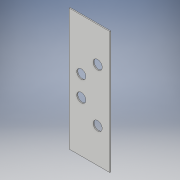
# Autodesk Inventor part: Holding Plate
Saved by Autodesk Inventor 2018 (Build 220112000, 112)
## iProperties
Created: 2019-01-15
Part Number: Holding Plate
Material: Generic
Document SubType Name: Modeling
Designer: Gabriel
Density: 1 g/cm^3
Appearance: Default
Author: Gabriel
Autodesk Inventor part; units mm, degrees
ref_plane "YZ Plane" through (0, 0, 0) normal (1, 0, 0) x (0, 1, 0)
ref_plane "XZ Plane" through (0, 0, 0) normal (0, 1, 0) x (-1, 0, 0)
ref_plane "XY Plane" through (0, 0, 0) normal (0, 0, 1) x (1, 0, 0)
sketch "Sketch1" plane through (0, 0, 0) normal (0, 0, 1) x (1, 0, 0)
  line L0 (-52.0393, 256.0699) -> (74.9607, 256.0699)
  line L1 (74.9607, 256.0699) -> (74.9607, -124.9301)
  line L2 (74.9607, -124.9301) -> (-52.0393, -124.9301)
  line L3 (-52.0393, -124.9301) -> (-52.0393, 256.0699)
  point P0 (0, 0)
  dimension "d0" = 127
  dimension "d1" = 381
  constraints: 8 end point, 2 parallel, 1 horizontal, 1 perpendicular
  measures "d0" distance of L1.end L2.end
  measures "d1" distance of L0.end L1.end
extrude "Extrusion1" add sketch "Sketch1" along normal blind 3.175
sketch "Sketch3" plane through (0, 0, 3.175) normal (0, 0, 1) x (1, 0, 0)
  line L0 (-52.0393, 256.0699) -> (-52.0393, -124.9301) projected
  line L1 (-52.0393, 65.5699) -> (-45.6893, 65.5699) construction
  line L2 (-45.6893, 65.5699) -> (-13.9457, 64.9297) construction
  line L3 (-13.9457, 64.9297) -> (-13.9457, 96.6797) construction
  line L4 (-13.9457, 64.9297) -> (17.8043, 64.9297) construction
  line L5 (-13.9457, 64.9297) -> (-13.9457, 33.1797) construction
  line L6 (-13.9457, 64.9297) -> (17.8043, 64.9297) construction
  line L7 (-13.9457, 96.6797) -> (36.8543, 96.6797) construction
  line L8 (36.8543, 96.6797) -> (36.8543, 147.4797) construction
  line L9 (36.8543, 147.4797) -> (-13.9457, 147.4797) construction
  line L10 (-13.9457, 147.4797) -> (-13.9457, 96.6797) construction
  circle A0 centre (36.8543, 147.4797) radius 14.2875
  line L11 (-13.9457, 33.1797) -> (36.8543, 33.1797) construction
  line L12 (36.8543, 33.1797) -> (36.8543, -17.6203) construction
  line L13 (36.8543, -17.6203) -> (-13.9457, -17.6203) construction
  line L14 (-13.9457, -17.6203) -> (-13.9457, 33.1797) construction
  circle A1 centre (36.8543, -17.6203) radius 14.2875
  circle A2 centre (-13.9457, 96.6797) radius 14.2875
  circle A3 centre (-13.9457, 33.1797) radius 14.2875
  dimension "d20" = 6.35
  dimension "d21" = 31.75
  dimension "d22" = 31.75
  dimension "d23" = 90
  dimension "d24" = 31.75
  dimension "d25" = 90
  dimension "d26" = 50.8
  dimension "d27" = 50.8
  dimension "d28" = 28.575
  dimension "d29" = 50.8
  dimension "d30" = 50.8
  dimension "d31" = 28.575
  dimension "d36" = 28.575
  dimension "d37" = 28.575
  constraints: 28 end point, 6 coincident, 5 horizontal, 4 centre point, 4 parallel, 4 perpendicular, 2 vertical, 1 midpoint
  measures "d20" distance of L1.start L1.end
  measures "d21" distance of L1.end L2.end
  measures "d22" distance of L2.end L3.end
  measures "d23" angle of L4 L3
  measures "d24" distance of L2.end L5.end
  measures "d25" angle of L5 L6
  measures "d26" distance of L9.end L8.end
  measures "d27" distance of L8.end L7.end
  measures "d28" diameter of A0
  measures "d29" distance of L12.end L13.end
  measures "d30" distance of L11.end L12.end
  measures "d31" diameter of A1
  measures "d36" diameter of A2
  measures "d37" diameter of A3
extrude "Extrusion2" cut sketch "Sketch3" against normal blind 25.4
body "Solid1"
